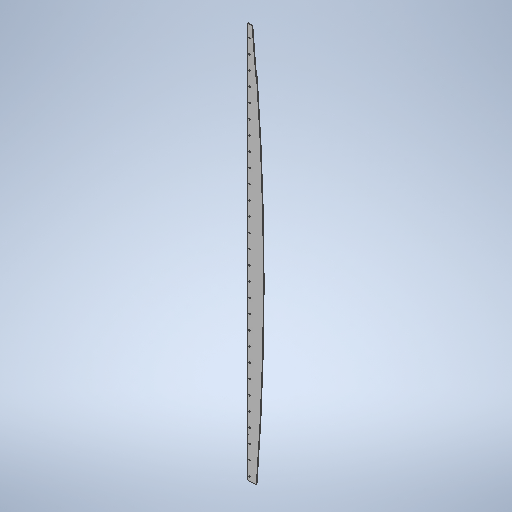
# Autodesk Inventor part: MSC 084 wall support gills
Saved by Autodesk Inventor 2025 (Build 290162010, 162A)
## iProperties
Created: 2024-04-18
Part Number: MSC 084 wall support gills
Material: AISI304
Document SubType Name: Sheet Metal
Designer: admin
Stock Number: МОО 084 стойка боковая жабры
Mass: 2923.41 g
Surface Area: 2574.94 cm^2
Volume: 365.426 cm^3
Density: 8 g/cm^3
Sheet Metal Rule: AISI304 3mm
Sheet Metal Width: 77,902 mm
Sheet Metal Length: 1970,000 mm
Sheet Metal Area: 153467,325 mm^2
Appearance: Default
Flat Pattern Width: 7.79022 cm
Flat Pattern Length: 197 cm
Flat Pattern Area: 1534.67 cm^2
Author: admin
Autodesk Inventor part; units mm, degrees
ref_plane "YZ Plane" through (0, 0, 0) normal (1, 0, 0) x (0, 1, 0)
ref_plane "XZ Plane" through (0, 0, 0) normal (0, 1, 0) x (-1, 0, 0)
ref_plane "XY Plane" through (0, 0, 0) normal (0, 0, 1) x (1, 0, 0)
sketch "Sketch1" plane through (0, 0, 0) normal (0, 0, 1) x (1, 0, 0)
  line L0 (0, 100) -> (0, 50) construction
  line L1 (0, 47) -> (0, 0) construction
  line L2 (0, 50) -> (0, 47) construction
  arc A0 (42, -1970) -> (25, 0) centre (-10972.0978, -1079.9722) ccw
  line L3 (42, -1970) -> (0, -1970)
  line L4 (0, -1970) -> (0, 0)
  line L5 (0, 0) -> (25, 0)
  line L6 (21, 0) -> (39.6023, -210)
  line L7 (39.6023, -210) -> (43.6023, -210)
  dimension "d115" = 3
  dimension "d131" = 11050
  dimension "d132" = 25
  dimension "d133" = 42
  dimension "d134" = 1970
  dimension "d145" = 4
  dimension "d146" = 210
  dimension "d147" = 4
  measures "d115" distance of L0.end L1.start
  measures "d131" radius of A0
  measures "d132" distance of L1.end L5.end
  measures "d133" distance of L3.start L3.end
  measures "d134" distance of L1.end L3.end
  measures "d145" distance of L6.end L7.end
  measures "d146" distance from line of L5 L6.end
  measures "d147" distance of L5.end L6.start
extrude "Plate3" add sketch "Sketch1" along normal blind 3 contours L3 L4 L5 L6 L7 A0
sketch "Sketch3" plane through (0, 0, 0) normal (0, 0, -1) x (-1, 0, 0)
  line L0 (0, 0) -> (0, -1970) projected
  line L1 (-21, 0) -> (0, 0) projected
  arc A0 (-43.6023, -210) -> (-42, -1970) centre (10972.0978, -1079.9722) ccw projected
  line L2 (0, -1970) -> (-42, -1970) projected
  circle A1 centre (-8, -1950) radius 3.5
  circle A2 centre (0, -1947.1277) radius 5
  circle A3 centre (0, -1947.1277) radius 12
  line L3 (-39.6023, -210) -> (-21, 0) projected
  line L4 (-43.6023, -210) -> (-39.6023, -210) projected
  point P0 (0, -1935.1277)
  point P1 (-11.2941, -1951.1827)
  point P2 (-4.7059, -1948.8173)
  point P3 (0, -1942.1277)
  dimension "d135" = 7
  dimension "d136" = 8
  dimension "d137" = 20
  dimension "d143" = 10
  constraints: 3 centre point, 2 tangent, 1 coincident, 1 point on line
  measures "d135" diameter of A1
  measures "d136" distance from line of L0 A1.centre
  measures "d137" distance from line of L2 A1.centre
  measures "d143" diameter of A2
extrude "Extrusion2" cut sketch "Sketch3" against normal blind 10 contours A1
pattern_linear "Rectangular Pattern1" count 31 spacing 70 along (0, 1, 0) of "Extrusion2"
equation "\"BendReliefWidth\" = Thickness"
equation "\"BendReliefDepth\" = 0.5 * Thickness"
equation "\"CornerReliefSize\" = 4 * Thickness"
equation "\"MinimumRemnant\" = 2 * Thickness"
equation "\"GapSize\" = Thickness"
equation "\"Thickness\" = 3"
body "Solid4"
